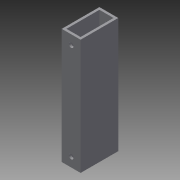
# Autodesk Inventor part: 2x1 axle support
Saved by Autodesk Inventor 2015 (Build 190159000, 159)
## iProperties
Created: 2015-01-22
Part Number: 2x1 axle support
Material: Generic
Document SubType Name: Modeling
Designer: 215152
Density: 1 g/cm^3
Appearance: Default
Author: 215152
Autodesk Inventor part; units mm, degrees
ref_plane "YZ Plane" through (0, 0, 0) normal (1, 0, 0) x (0, 1, 0)
ref_plane "XZ Plane" through (0, 0, 0) normal (0, 1, 0) x (-1, 0, 0)
ref_plane "XY Plane" through (0, 0, 0) normal (0, 0, 1) x (1, 0, 0)
sketch "Sketch1" plane through (0, 0, 0) normal (0, 1, 0) x (-1, 0, 0)
  line L0 (0, 0) -> (25.4, 0)
  line L1 (25.4, 0) -> (25.4, 50.8)
  line L2 (25.4, 50.8) -> (0, 50.8)
  line L3 (0, 50.8) -> (0, 0)
  line L4 (3.175, 3.175) -> (22.225, 3.175)
  line L5 (22.225, 3.175) -> (22.225, 47.625)
  line L6 (22.225, 47.625) -> (3.175, 47.625)
  line L7 (3.175, 47.625) -> (3.175, 3.175)
  dimension "d0" = 25.4
  dimension "d1" = 50.8
  dimension "d2" = 19.05
  dimension "d3" = 44.45
  dimension "d4" = 3.175
  dimension "d5" = 3.175
  constraints: 16 end point, 4 parallel, 2 horizontal, 2 perpendicular
  measures "d0" distance of L2.end L1.end
  measures "d1" distance of L1.end L0.end
  measures "d2" distance of L6.end L5.end
  measures "d3" distance of L5.end L4.end
  measures "d4" distance between parallel lines of L3 L7
  measures "d5" distance between parallel lines of L0 L4
extrude "Extrusion1" add sketch "Sketch1" along normal blind 155.575
sketch "Sketch2" plane through (-25.4, 0, 50.8) normal (0, 0, 1) x (1, 0, 0)
  line L0 (0, 0) -> (25.4, 0) projected
  line L1 (25.4, 0) -> (25.4, 155.575) projected
  line L2 (0, 155.575) -> (25.4, 155.575) projected
  line L3 (0, 0) -> (0, 155.575) projected
  point P0 (12.7, 142.875)
  point P1 (12.7, 12.7)
  dimension "d8" = 12.7
  dimension "d9" = 12.7
  dimension "d10" = 12.7
  dimension "d11" = 12.7
  measures "d8" distance from line of L0 point (12.7, 12.7)
  measures "d9" distance from line of L3 point (12.7, 12.7)
  measures "d10" distance from line of L3 point (12.7, 142.875)
  measures "d11" distance from line of L2 point (12.7, 142.875)
hole "Hole1" at (-12.7, 142.875, 50.8) at (-12.7, 12.7, 50.8) direction (0, 0, -1) diameter 6.35 end through all
sketch "Sketch3" plane through (-25.4, 0, 0) normal (-1, 0, 0) x (0, 0, 1)
  line L0 (0, 0) -> (50.8, 0) projected
  line L1 (50.8, 0) -> (50.8, 155.575) projected
  line L2 (0, 155.575) -> (50.8, 155.575) projected
  line L3 (0, 0) -> (0, 155.575) projected
  circle A0 centre (41.275, 85.725) radius 4.7625 construction
  line L4 (41.275, 85.725) -> (41.275, 80.9625) construction
  line L5 (41.275, 85.725) -> (41.275, 90.4875) construction
  line L6 (50.8, 90.4875) -> (41.275, 90.4875)
  line L7 (50.8, 0) -> (50.8, 155.575) projected
  line L8 (50.8, 80.9625) -> (41.275, 80.9625)
  line L9 (50.8, 90.4875) -> (50.8, 80.9625)
  arc A1 (41.275, 90.4875) -> (41.275, 80.9625) centre (41.275, 85.725) ccw
  dimension "d19" = 85.725
  dimension "d20" = 9.525
  dimension "d21" = 9.525
  constraints: 10 end point, 4 point on circle, 4 tangent, 2 centre point, 2 point on line, 2 vertical, 1 coincident, 1 collinear, 1 horizontal, 1 perpendicular
  measures "d19" distance from line of L0 point (41.275, 85.725)
  measures "d20" distance from line of L1 point (41.275, 85.725)
  measures "d21" diameter of A0
extrude "Extrusion2" cut sketch "Sketch3" against normal blind 155.575 contours L8 A1 L6 L1
body "Solid1"
